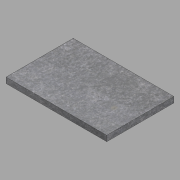
# Autodesk Inventor part: 24x36x2-50
Saved by Autodesk Inventor 2022.2 (Build 262287000, 287)
## iProperties
Created: 2022-02-10
Part Number: 24x36x2-50
Material: Granite, Cut, Polished
Document SubType Name: Modeling
Designer: awelt
Density: 2.7 g/cm^3
Appearance: Kasota SN sapphire
Author: awelt
Autodesk Inventor part; units mm, degrees
ref_plane "YZ Plane" through (0, 0, 0) normal (1, 0, 0) x (0, 1, 0)
ref_plane "XZ Plane" through (0, 0, 0) normal (0, 1, 0) x (-1, 0, 0)
ref_plane "XY Plane" through (0, 0, 0) normal (0, 0, 1) x (1, 0, 0)
sketch "Sketch3" plane through (0, 0, 0) normal (0, 1, 0) x (-1, 0, 0)
  line L0 (457.2, -304.8) -> (-457.2, -304.8)
  line L1 (-457.2, -304.8) -> (-457.2, 304.8)
  line L2 (-457.2, 304.8) -> (457.2, 304.8)
  line L3 (457.2, 304.8) -> (457.2, -304.8)
  line L4 (457.2, -304.8) -> (-457.2, 304.8) construction
  line L5 (-457.2, -304.8) -> (457.2, 304.8) construction
  point P0 (0, 0)
  dimension "d4" = 914.4
  dimension "d5" = 609.6
  constraints: 12 end point, 2 midpoint, 2 parallel, 1 horizontal, 1 perpendicular
  measures "d4" distance of L1.end L2.end
  measures "d5" distance of L0.end L1.end
extrude "Extrusion2" add sketch "Sketch3" along normal blind 50.8
body "Solid2"
